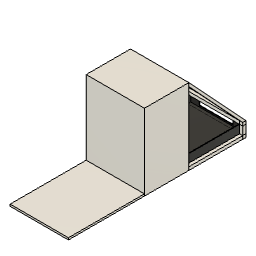
2023-12-18-3d (Autodesk Fusion 360 design; units mm, degrees)
Autodesk Fusion 360 part; units mm, degrees
note: some values were not read from the file. Set by a fixed rule: which face or edge a step refers to.
sketch "Esquisse1" plane through (0, 0, 0) normal (0, 0, 1) x (1, 0, 0)
  line L0 (-46, 0) -> (46, 0)
  line L1 (46, 0) -> (46, 120)
  line L2 (46, 120) -> (-46, 120)
  line L3 (-46, 120) -> (-46, 0)
  dimension "d1" = 92
  dimension "d2" = 120
  constraint horizontal L0
  constraint vertical L1
  constraint horizontal L2
  constraint vertical L3
  constraint midpoint L0 origin
  measures "d1" distance of L0.start L0.end
  measures "d2" distance of L0.start L2.end
extrude "Extrusion1" add sketch "Esquisse1" along normal blind 70 makes body 1
shell "Coque1" thickness 5 removed faces 1 at (-15.3333, 80, 0) on bodies 1
sketch "Esquisse2" plane through (-46, 0, 0) normal (-1, 0, 0) x (0, 0, 1)
  line L0 (0, 120) -> (0, 0)
  line L1 (0, 0) -> (70, 0)
  line L2 (70, 0) -> (70, 120)
  line L3 (70, 120) -> (0, 120)
  line L4 (0, 0) -> (-90, 0)
  line L5 (-90, 0) -> (-90, 5)
  line L6 (-90, 5) -> (0, 5)
  line L7 (0, 5) -> (0, 0)
  line L8 (-90, 0) -> (-85, 0)
  line L9 (-90, 5) -> (-85, 5)
  line L10 (-85, 5) -> (-85, 23)
  line L11 (-85, 23) -> (-90, 23)
  line L12 (-90, 23) -> (-90, 5)
  line L13 (-90, 23) -> (0, 120)
  line L14 (-90, 23) -> (-85, 23)
  line L15 (-85, 23) -> (0, 114.6111)
  line L16 (0, 114.6111) -> (0, 120)
  dimension "d6" = 90
  dimension "d7" = 5
  dimension "d8" = 5
  dimension "d28" = 5
  dimension "d29" = 18
  constraint horizontal L4
  constraint vertical L5
  constraint horizontal L6
  constraint vertical L7
  constraint coincident L0.end L1.start
  constraint horizontal L8
  constraint horizontal L9
  constraint vertical L10
  constraint horizontal L11
  constraint vertical L12
  constraint coincident L0 L15.end
  constraint parallel L13 L15
  constraint coincident L0.start L3.end
  constraint perpendicular L3 L16
  measures "d6" distance of L0.end L4.end
  measures "d7" distance of L0.end L6.end
  measures "d8" distance of L4.end L8.end
  measures "d28" distance of L5.end L9.end
  measures "d29" distance of L5.end L11.end
sketch "Esquisse4" plane through (0, 120, 0) normal (0, 1, 0) x (-1, 0, 0)
  line L0 (-46, 0) -> (46, 0)
  line L1 (46, 0) -> (46, 70)
  line L2 (46, 70) -> (-46, 70)
  line L3 (-46, 70) -> (-46, 0)
  line L4 (-46, 0) -> (46, 0)
  line L5 (46, 0) -> (46, -5)
  line L6 (46, -5) -> (-46, -5)
  line L7 (-46, -5) -> (-46, 0)
  dimension "d12" = 92
  dimension "d13" = 5
  constraint horizontal L4
  constraint vertical L5
  constraint horizontal L6
  constraint vertical L7
  constraint coincident L0.start L3.end
  measures "d12" distance of L0.start L0.end
  measures "d13" distance of L0.start L6.end
extrude "Extrusion3" add sketch "Esquisse4" along normal blind 5 separate body contours L0 L4 L5 L6 L7 makes body 2
move_body "Déplacer3" bodies 2 to x (1, 0, 0) y (0, 1, 0) z (0, 0, 1) at (0, -5, 0)
move_body "Déplacer4" bodies 2 to x (1, 0, 0) y (0, 1, 0) z (0, 0, 1) at (0, -115, 0)
move_body "Déplacer5" bodies 2 to x (1, 0, 0) y (0, 1, 0) z (0, 0, 1) at (0, 0, -85)
copy_body "Copier/Coller des corps2" bodies 2 makes body 3
move_body "Déplacer6" bodies 3 to x (1, 0, 0) y (0, 1, 0) z (0, 0, 1) at (0, 13, 0)
sketch "Esquisse5" plane through (0, 120, 0) normal (0, 1, 0) x (-1, 0, 0)
  line L0 (-46, 0) -> (46, 0)
  line L1 (46, 0) -> (46, 70)
  line L2 (46, 70) -> (-46, 70)
  line L3 (-46, 70) -> (-46, 0)
  line L4 (0, 0) -> (-92, 0)
  line L5 (-92, 0) -> (-92, 120)
  line L6 (-92, 120) -> (0, 120)
  line L7 (0, 120) -> (0, 0)
  dimension "d16" = 92
  dimension "d17" = 120
  constraint horizontal L4
  constraint vertical L5
  constraint horizontal L6
  constraint vertical L7
  constraint coincident L4.start L7.end
  measures "d16" distance of L4.start L4.end
  measures "d17" distance of L4.start L6.end
extrude "Extrusion4" add sketch "Esquisse5" along normal blind 3 separate body contours L0 L2 L3 L4 L7 | L2 L3 L4 L5 L6 L7 makes body 4
move_body "Déplacer7" bodies 4 to x (1, 0, 0) y (0, 1, 0) z (0, 0, 1) at (0, -120, 0)
move_body "Déplacer8" bodies 4 to x (1, 0, 0) y (0, 1, 0) z (0, 0, 1) at (-46, 0, 0)
move_body "Déplacer9" bodies 4 to x (1, 0, 0) y (0, 1, 0) z (0, 0, 1) at (0, 0, 70)
move_body "Déplacer14" bodies 3 to x (1, 0, 0) y (0, 1, 0) z (0, 0, 1) at (0, 5, 0)
extrude "Extrusion7" add sketch "Esquisse2" along normal blind 5 separate body contours L0 L11 L13 L14 L15 L16 | L6 L9 L10 L11 L12 L14 | L0 L4 L5 L6 L7 L8 L9 makes body 5
copy_body "Copier/Coller des corps3" bodies 5 makes body 6
move_body "Déplacer15" bodies 6 to x (1, 0, 0) y (0, 1, 0) z (0, 0, 1) at (5, 0, 0)
move_body "Déplacer16" bodies 5 to x (1, 0, 0) y (0, 1, 0) z (0, 0, 1) at (92, 0, 0)
sketch "Esquisse8" plane through (0, 0, 0) normal (0, 0, 1) x (1, 0, 0)
  line L0 (0, 0) -> (-53.34, 0)
  line L1 (-53.34, 0) -> (-53.34, 10)
  line L2 (-53.34, 10) -> (0, 10)
  line L3 (0, 10) -> (0, 0)
  point P0 (-26.67, 0)
  dimension "d33" = 53.34
  dimension "d34" = 10
  constraint coincident L0.start L3.end
  constraint midpoint L0 P0
  measures "d33" distance of L0.start L0.end
  measures "d34" distance of L0.start L2.end
sketch "Esquisse9" plane through (0, 120, 0) normal (0, 1, 0) x (-1, 0, 0)
  line L0 (-46, 0) -> (46, 0)
  line L1 (46, 0) -> (46, 70)
  line L2 (46, 70) -> (-46, 70)
  line L3 (-46, 70) -> (-46, 0)
  line L4 (-46, 70) -> (36, 70)
  line L5 (36, 70) -> (36, -85)
  line L6 (36, -85) -> (-46, -85)
  line L7 (-46, -85) -> (-46, 70)
  dimension "d37" = 82
  dimension "d38" = 155
  constraint horizontal L4
  constraint vertical L5
  constraint horizontal L6
  constraint vertical L7
  constraint coincident L2.end L3.start
  measures "d37" distance of L2.end L4.end
  measures "d38" distance of L2.end L6.end
extrude "Extrusion9" add sketch "Esquisse9" along normal blind 13 separate body contours L0 L2 L3 L4 L5 L7 | L0 L5 L6 L7 makes body 7
move_body "Déplacer20" bodies 7 to x (1, 0, 0) y (0, 1, 0) z (0, 0, 1) at (-5, 0, 0)
move_body "Déplacer21" bodies 7 to x (1, 0, 0) y (0, 1, 0) z (0, 0, 1) at (0, -115, 0)
move_body "Déplacer22" bodies 7 to x (1, 0, 0) y (0, 1, 0) z (0, 0, 1) at (0, 0, -5)
shell "Coque3" thickness 1 removed faces 1 at (13.6667, 18, -61.6667) on bodies 7
sketch "Esquisse14" plane through (0, 0, 0) normal (0, 0, 1) x (1, 0, 0)
  line L0 (26.7945, 19.184) -> (26.7945, 7.9226)
  line L1 (26.7945, 7.9226) -> (-26.6055, 7.9226)
  line L2 (-26.6055, 7.9226) -> (-26.6055, 19.4429)
  dimension "d48" = 53.4
  constraint vertical L0
  constraint perpendicular L0 L1
  constraint perpendicular L1 L2
  measures "d48" distance of L0.end L1.end
split_face "ScinderLesFaces1" 1 faces at (-13.6667, 13.6667, -90) by curves path "Esquisse14" along L0 L1 L2 on bodies 7
extrude "Extrusion10" cut 1 faces at (-8.8055, 11.2817, -90) along direction (0, 0, 1) blind 60 on bodies 7 bodies 7
named bodies: "structure_avant", "front_panel"
